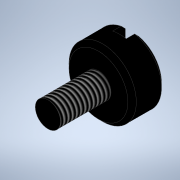
# Autodesk Inventor part: CSMKN-SUSTBS-M3-6
Saved by Autodesk Inventor 2022.3 (Build 263350000, 350)
## iProperties
Part Number: CSMKN-SUSTBS-M3-6
Material: ステンレス鋼 AISI 304
Document SubType Name: Modeling
Designer: Masato Kubotera
Density: 8.79216 g/cm^3
Appearance: 陽極酸化 - 黒
Mass: 2.5 g
Surface Area: 2.61352 cm^2
Volume: 0.218784 cm^3
Description: ReadyMade
Catalog Web Link: https://jp.misumi-ec.com/vona2/detail/221000545975/?HissuCode=CSMKN-SUSTBS-M3-6
Author: Masato Kubotera
Autodesk Inventor part; units mm, degrees
ref_plane "YZ Plane" through (0, 0, 0) normal (1, 0, 0) x (0, 1, 0)
ref_plane "XZ Plane" through (0, 0, 0) normal (0, 1, 0) x (-1, 0, 0)
ref_plane "XY Plane" through (0, 0, 0) normal (0, 0, 1) x (1, 0, 0)
sketch "スケッチ1" plane through (0, 0, 0) normal (0, 1, 0) x (-1, 0, 0)
  line L0 (0, 0) -> (0, 10)
  line L1 (0, 0) -> (3.5, 0)
  line L2 (4, 0.5) -> (4, 3.5)
  line L3 (3.5, 4) -> (1.5, 4)
  line L4 (1.5, 4) -> (1.5, 10)
  line L5 (1.5, 10) -> (0, 10)
  line L6 (-0.8, 1.5) -> (0.8, 1.5)
  line L7 (0.8, 1.5) -> (0.8, 0)
  line L8 (0.8, 0) -> (-0.8, 0)
  line L9 (-0.8, 0) -> (-0.8, 1.5)
  line L10 (-0.8, 1.5) -> (0.8, 0) construction
  line L11 (0.8, 1.5) -> (-0.8, 0) construction
  line L12 (3.5, 0) -> (4, 0.5)
  line L13 (4, 3.5) -> (3.5, 4)
  point P0 (4, 0)
  point P1 (4, 4)
  point P2 (0, 0.75)
  dimension "d7" = 4
  dimension "d8" = 6
  dimension "d12" = 3
  dimension "d13" = 8
  dimension "d20" = 1.5
  dimension "d21" = 1.6
  dimension "d24" = 0.5
  dimension "d25" = 0.5
  dimension "d26" = 0.5
  dimension "d27" = 0.5
  constraints: 28 end point, 5 point on line, 4 perpendicular, 3 midpoint, 2 horizontal, 2 parallel, 1 vertical
  measures "d7" distance of point (4, 0) point (4, 4)
  measures "d8" distance of L3.end L4.end
  measures "d12" diameter of L4 L0
  measures "d13" diameter of L2 L0
  measures "d20" distance of L6.end L7.end
  measures "d21" distance of L7.end L8.end
  measures "d24" distance of L1.end point (4, 0)
  measures "d25" distance of L2.start point (4, 0)
  measures "d26" distance of L2.end point (4, 4)
  measures "d27" distance of L3.start point (4, 4)
revolve "回転1" add sketch "スケッチ1" angle 360 about axis through (0, 0, 0) along (0, 0, 1) contours L0 L6 L7 L1 | L0 L5 L4 L3 L13 L2 L12 L1 L7 L6
thread "ねじ1" size "M3x0.5" class "6g" standard "ANSI Metric M Profile" full length
extrude "押し出し1" cut sketch "スケッチ1" along normal through all both and the other way through all contours L8 L9 L6 L0 | L0 L6 L7 L1
equation "\"d25\" = d24"
equation "\"d26\" = d24"
equation "\"d27\" = d26"
